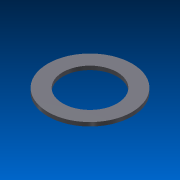
# Autodesk Inventor part: 12mm Incremental Encoder Washer
Saved by Autodesk Inventor 2014 (Build 180170000, 170)
## iProperties
Created: 2011-11-07
Part Number: 12mm Incremental Encoder Washer
Document SubType Name: Modeling
Designer: sdarley
Density: 1 g/cm^3
Material: Generic
Appearance: Steel - Polished
Author: sdarley
Autodesk Inventor part; units mm, degrees
ref_plane "YZ Plane" through (0, 0, 0) normal (1, 0, 0) x (0, 1, 0)
ref_plane "XZ Plane" through (0, 0, 0) normal (0, 1, 0) x (-1, 0, 0)
ref_plane "XY Plane" through (0, 0, 0) normal (0, 0, 1) x (1, 0, 0)
sketch "Sketch1" plane through (0, 0, 0) normal (0, 0, 1) x (1, 0, 0)
  circle A0 centre (-6.425, 0) radius 2 projected
  circle A1 centre (-6.425, 0) radius 5.5
  circle A2 centre (-6.425, 0) radius 3.55
  point P0 (0, 0)
  dimension "d0" = 11
  dimension "d1" = 7.1
  constraints: 2 centre point, 2 coincident
  measures "d0" diameter of A1
  measures "d1" diameter of A2
extrude "Extrusion1" add sketch "Sketch1" along normal blind 0.5 contours A1
body "Solid1"
